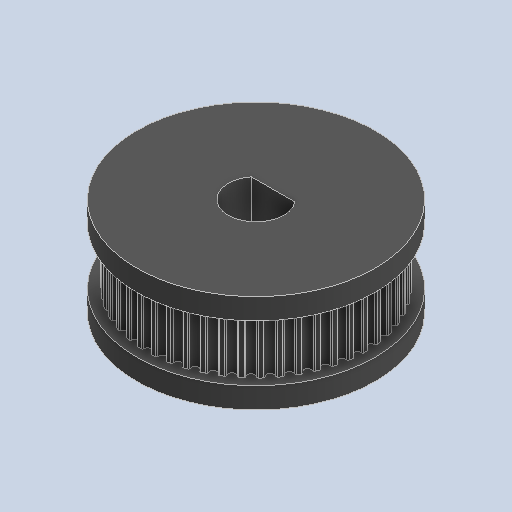
# Autodesk Inventor part: Engranaje GT2 Parametrico
Saved by Autodesk Inventor 2026 (Build 300175050, 175E)
## iProperties
Created: 2025-07-19
Part Number: Engranaje GT2 Parametrico
Material: Plastico PETG
Document SubType Name: Modeling
Designer: bello
Density: 1.27 g/cm^3
Appearance: Genérico
Author: bello
Autodesk Inventor part; units mm, degrees
ref_plane "YZ Plane" through (0, 0, 0) normal (1, 0, 0) x (0, 1, 0)
ref_plane "XZ Plane" through (0, 0, 0) normal (0, 1, 0) x (-1, 0, 0)
ref_plane "XY Plane" through (0, 0, 0) normal (0, 0, 1) x (1, 0, 0)
sketch "Boceto1" plane through (0, 0, 0) normal (0, 1, 0) x (-1, 0, 0)
  circle A0 centre (0, 0) radius 15.661494
  circle A1 centre (0, 0) radius 14.911494
  line L0 (0, 0) -> (0, -15.661494)
  line L1 (0, 0) -> (-1.962906, -15.537999)
  circle A2 centre (0, -15.466494) radius 0.555
  circle A3 centre (-1.938466, -15.344536) radius 0.555
  circle A4 centre (-0.704403, -15.495492) radius 0.15
  circle A5 centre (-1.243251, -15.461591) radius 0.15
  circle A6 centre (0, 0) radius 12.911494
  point P0 (0, -12.911494)
  point P1 (-1.618239, -12.809683)
  point P2 (-1.868906, -14.793913)
  point P3 (-1.391169, -15.436685)
  point P4 (-1.255274, -15.611108)
  point P5 (-0.711215, -15.645337)
  point P6 (-0.55453, -15.489322)
  point P7 (0, -14.911494)
  dimension "d0" = 31.32299
  dimension "d1" = 29.82299
  dimension "d2" = 7.2
  dimension "d3" = 1.11
  dimension "d4" = 0.3
  dimension "d5" = 25.82299
  constraints: 7 centre point, 6 tangent, 4 end point, 3 coincident, 2 equal radius, 2 point on circle, 2 point on line, 1 vertical
  measures "d0" diameter of A0
  measures "d1" diameter of A1
  measures "d2" angle of L0 L1
  measures "d3" diameter of A2
  measures "d4" diameter of A4
  measures "d5" diameter of A6
sketch "Boceto1 outline for Extrusión1" plane through (0, 0, 0) normal (0, 1, 0) x (-1, 0, 0)
  line L0 (0, -14.911494) -> (0, 0)
  line L1 (0, 0) -> (-1.868906, -14.793913)
  arc A0 (-1.868906, -14.793913) -> (-1.391169, -15.436685) centre (-1.938466, -15.344536) cw
  arc A1 (-1.391169, -15.436685) -> (-1.255274, -15.611108) centre (-1.243251, -15.461591) ccw
  arc A2 (-1.255274, -15.611108) -> (-0.711215, -15.645337) centre (0, 0) ccw
  arc A3 (-0.711215, -15.645337) -> (-0.55453, -15.489322) centre (-0.704403, -15.495492) ccw
  arc A4 (-0.55453, -15.489322) -> (0, -14.911494) centre (0, -15.466494) cw
extrude "Extrusión1" add sketch "Boceto1 outline for Extrusión1" along normal blind 8
pattern_circular "Patrón circular1" count 50 over 360 about axis through (0, -10, 0) along (0, 1, 0) of "Extrusión1"
sketch "Boceto2" plane through (0, 8, 0) normal (0, 1, 0) x (1, 0, 0)
  circle A0 centre (0, 0) radius 17
  dimension "d11" = 34
  constraints: 1 centre point, 1 coincident
  measures "d11" diameter of A0
extrude "Extrusión2" add sketch "Boceto2" along normal blind 3
sketch "Boceto3" plane through (0, 0, 0) normal (0, -1, 0) x (1, 0, 0)
  circle A0 centre (0, 0) radius 17
  dimension "d27" = 34
  constraints: 1 centre point, 1 coincident
  measures "d27" diameter of A0
extrude "Extrusión3" add sketch "Boceto3" along normal blind 3
sketch "Boceto8" plane through (0, 11, 0) normal (0, 1, 0) x (1, 0, 0)
  circle A0 centre (0, 0) radius 3.95
  line L0 (-7.227451, 2.45) -> (7.535341, 2.45)
  line L1 (0, -3.95) -> (7.535341, -3.95)
  point P0 (3.098387, 2.45)
  point P1 (-3.098387, 2.45)
  dimension "d32" = 7.9
  dimension "d33" = 6.4
  constraints: 4 end point, 3 horizontal, 1 coincident, 3 other
  measures "d33" distance between parallel lines of L1 L0
extrude "Extrusión6" cut sketch "Boceto8" against normal through all contours A0 L0 picked at (-0.324311, 0.357233)
equation "\"d0\" = PitchDiameter"
equation "\"d1\" = InnerDiameter"
equation "\"d2\" = ToothAngle"
equation "\"d3\" = RootDiameter"
equation "\"d4\" = ShoulderDiameter"
equation "\"Pitch\" = 2"
equation "\"InnerDiameter\" = PitchDiameter - 2 * ToothHeight"
equation "\"PitchDiameter\" = PulleyDiameter - 2 * PLD"
equation "\"PLD\" = 0.254"
equation "\"ToothHeight\" = 0.75"
equation "\"ShoulderDiameter\" = 0.3"
equation "\"RootDiameter\" = 1.11"
equation "\"ToothAngle\" = 7.2deg"
equation "\"PulleyDiameter\" = 31.830989"
